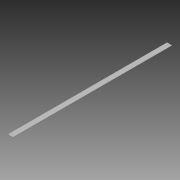
# Autodesk Inventor part: 2p6fs1
Saved by Autodesk Inventor 2014 (Build 180170000, 170)
## iProperties
Company: HERA Project
Created: 2013-12-11
Part Number: 2p6fs1
Material: Steel
Document SubType Name: Modeling
Designer: David DeBoer
Mass: 925.881 g
Surface Area: 993.091 cm^2
Volume: 117.947 cm^3
Density: 7.85 g/cm^3
Description: inner furring strip
Appearance: Steel
Author: David DeBoer
Autodesk Inventor part; units mm, degrees
ref_plane "YZ Plane" through (0, 0, 0) normal (1, 0, 0) x (0, 1, 0)
ref_plane "XZ Plane" through (0, 0, 0) normal (0, 1, 0) x (-1, 0, 0)
ref_plane "XY Plane" through (0, 0, 0) normal (0, 0, 1) x (1, 0, 0)
sketch "Sketch1" plane through (0, 0, 0) normal (0, 0, 1) x (1, 0, 0)
  line L0 (0, 0) -> (38.1, 0)
  line L1 (38.1, 0) -> (38.1, 2.54)
  line L2 (38.1, 2.54) -> (0, 2.54)
  line L3 (0, 2.54) -> (0, 0)
  dimension "d0" = 38.1
  dimension "d1" = 2.54
  constraints: 8 end point, 2 parallel, 1 horizontal, 1 perpendicular
  measures "d0" distance of L0.start L0.end
  measures "d1" distance of L2.end L0.start
extrude "Extrusion1" add sketch "Sketch1" along normal blind 1219.2
sketch "Sketch2" plane through (0, 2.54, 0) normal (0, 1, 0) x (1, 0, 0)
  line L0 (38.1, 0) -> (0, 0) projected
  circle A0 centre (19.05, -12.7) radius 2.2451
  dimension "d4" = 12.7
  constraints: 1 centre point
  measures "d4" distance from line of A0.centre L0
hole "Hole1" at (19.05, 2.54, 12.7) direction (0, -1, 0) diameter 3.175 end through all
sketch "Sketch3" plane through (0, 2.54, 0) normal (0, 1, 0) x (1, 0, 0)
  line L0 (38.1, -1219.2) -> (0, -1219.2) projected
  circle A0 centre (19.05, -1206.5) radius 2.2451
  dimension "d12" = 12.7
  constraints: 1 centre point
  measures "d12" distance from line of L0 A0.centre
hole "Hole2" at (19.05, 2.54, 1206.5) direction (0, -1, 0) diameter 3.175 end through all
body "Solid1"
